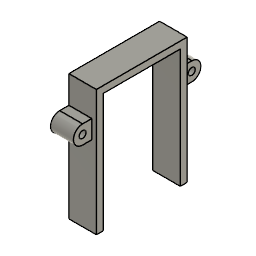
AG05 (Autodesk Fusion 360 design; units mm, degrees)
part number: 2025-10-09-12-51-14-243
Autodesk Fusion 360 part; units mm, degrees
note: some values were not read from the file. Set by a fixed rule: which sketch regions a step uses.
sketch "Boceto1" plane through (0, 0, 0) normal (0, 0, 1) x (1, 0, 0)
  line L0 (-38.0232, 20.8447) -> (47.9768, 20.8447)
  line L1 (47.9768, 20.8447) -> (47.9768, -12.6553)
  line L2 (47.9768, -12.6553) -> (-38.0232, -12.6553)
  line L3 (-38.0232, -12.6553) -> (-38.0232, 20.8447)
  line L4 (-41.0232, 23.8447) -> (50.9768, 23.8447)
  line L5 (50.9768, -15.6553) -> (-41.0232, -15.6553)
  line L6 (-38.0232, 20.8447) -> (-41.0232, 20.8447)
  line L7 (-41.0232, 20.8447) -> (50.9768, 20.8447)
  line L8 (-38.0232, -12.6553) -> (-41.0232, -12.6553)
  line L9 (-41.0232, -15.6553) -> (-41.0232, -12.6553)
  line L10 (-41.0232, 20.8447) -> (-41.0232, 23.8447)
  line L11 (47.9768, -12.6553) -> (50.9768, -12.6553)
  line L12 (50.9768, 23.8447) -> (50.9768, 20.8447)
  line L13 (50.9768, -12.6553) -> (50.9768, -15.6553)
  dimension "d1" = 86
  dimension "d2" = 33.5
  dimension "d3" = 3
  dimension "d4" = 3
  dimension "d5" = 3
  dimension "d6" = 3
  constraint horizontal L0
  constraint vertical L1
  constraint horizontal L2
  constraint vertical L3
  constraint horizontal L4
  constraint vertical L12
  constraint horizontal L5
  constraint vertical L9
  constraint coincident L6.end L9
  constraint perpendicular L6 L9
  constraint perpendicular L7 L12
  constraint perpendicular L8 L9
  constraint collinear L9 L10
  constraint coincident L11.end L12
  constraint perpendicular L11 L12
  constraint collinear L12 L13
  measures "d1" distance of L0.start L0.end
  measures "d2" distance of L0.end L1.end
  measures "d3" distance of L0 L4
  measures "d4" distance of L1 L12
  measures "d5" distance of L2 L5
  measures "d6" distance of L3 L9
extrude "Extruir1" add sketch "Boceto1" along normal blind 51 contours L0 L4 L6 L7 L10 L12 | L2 L5 L8 L9 L11 L13 makes body 1 at (20.3102, 20.8447, 17) makes body 2 at (20.3102, -12.6553, 17)
sketch "Boceto2" plane through (0, 0, 51) normal (0, 0, 1) x (-1, 0, 0)
  line L0 (41.0232, -20.8447) -> (-50.9768, -20.8447)
  line L1 (-50.9768, -20.8447) -> (-50.9768, -23.8447)
  line L2 (-50.9768, -23.8447) -> (41.0232, -23.8447)
  line L3 (41.0232, -23.8447) -> (41.0232, -20.8447)
  line L4 (41.0232, -23.8447) -> (-50.9768, -23.8447)
  line L5 (-50.9768, -23.8447) -> (-50.9768, 15.6553)
  line L6 (-50.9768, 15.6553) -> (41.0232, 15.6553)
  line L7 (41.0232, 15.6553) -> (41.0232, -23.8447)
  dimension "d9" = 39.5
  dimension "d12" = 92
  constraint horizontal L4
  constraint vertical L5
  constraint horizontal L6
  constraint vertical L7
  constraint coincident L2.end L3.start
  measures "d9" distance of L1.end L5.end
  measures "d12" distance of L5 L7
extrude "Extruir2" add sketch "Boceto2" along normal blind 3 bodies 1 2
sketch "Boceto3" plane through (0, 0, 51) normal (0, 0, -1) x (1, 0, 0)
  line L0 (-41.0232, -20.8447) -> (50.9768, -20.8447)
  line L1 (50.9768, -20.8447) -> (50.9768, 12.6553)
  line L2 (50.9768, 12.6553) -> (-41.0232, 12.6553)
  line L3 (-41.0232, 12.6553) -> (-41.0232, -20.8447)
  line L4 (50.9768, 12.6553) -> (47.9768, 12.6553)
  line L5 (47.9768, 12.6553) -> (47.9768, 5.6553)
  line L6 (47.9768, 5.6553) -> (50.9768, 5.6553)
  line L7 (50.9768, 5.6553) -> (50.9768, 12.6553)
  line L8 (50.9768, -20.8447) -> (47.9768, -20.8447)
  line L9 (47.9768, -20.8447) -> (47.9768, -13.8447)
  line L10 (47.9768, -13.8447) -> (50.9768, -13.8447)
  line L11 (50.9768, -13.8447) -> (50.9768, -20.8447)
  dimension "d13" = 3
  dimension "d14" = 3
  dimension "d16" = 7
  dimension "d17" = 7
  constraint horizontal L4
  constraint vertical L5
  constraint horizontal L6
  constraint vertical L7
  constraint coincident L1.end L2.start
  constraint horizontal L8
  constraint vertical L9
  constraint horizontal L10
  constraint vertical L11
  constraint coincident L0.end L1.start
  measures "d13" distance of L5 L7
  measures "d14" distance of L9 L11
  measures "d16" distance of L4.end L5.end
  measures "d17" distance of L0.end L10.end
extrude "Extruir3" add sketch "Boceto3" along normal blind 51 contours L0 L1 L8 L9 L10 L11 | L1 L2 L4 L5 L6 L7 bodies 1
extrude "Extruir4" cut 1 faces at (50.9768, -12.322, 35) along direction (-1, 0, 0) blind 80 on bodies 1 bodies 1
extrude "Extruir5" add 2 faces at (-37.0232, -14.6553, 0) (-37.0232, 22.8447, 0) along direction (0, 0, -1) blind 0.75 on bodies 1 bodies 1
sketch "Boceto4" plane through (0, 0, -0.75) normal (0, 0, -1) x (1, 0, 0)
  line L0 (-29.0232, -23.8447) -> (-29.0232, -20.8447)
  line L1 (-29.0232, -20.8447) -> (-41.0232, -20.8447)
  line L2 (-41.0232, -20.8447) -> (-41.0232, -23.8447)
  line L3 (-41.0232, -23.8447) -> (-29.0232, -23.8447)
  line L4 (-35.0232, -23.8447) -> (-35.0232, -27.8447) construction
  dimension "d24" = 4
  constraint midpoint L3 L4.start
  constraint perpendicular L3 L4
  measures "d24" distance of L4.start L4.end
sketch "Boceto5" plane through (-41.0232, 0, 0) normal (-1, 0, 0) x (0, -1, 0)
  line L0 (-20.8447, -0.75) -> (-20.8447, 51)
  line L1 (-20.8447, 51) -> (12.6553, 51)
  line L2 (12.6553, 51) -> (12.6553, -0.75)
  line L3 (12.6553, -0.75) -> (15.6553, -0.75)
  line L4 (15.6553, -0.75) -> (15.6553, 54)
  line L5 (15.6553, 54) -> (-23.8447, 54)
  line L6 (-23.8447, 54) -> (-23.8447, -0.75)
  line L7 (-23.8447, -0.75) -> (-20.8447, -0.75)
  line L8 (15.6553, -0.75) -> (15.6553, 51) construction
  line L9 (12.6553, -0.75) -> (-20.8447, -0.75) construction
  line L10 (-4.0947, -0.75) -> (-4.0947, 51) construction
  line L11 (-4.0947, 25.125) -> (-4.0947, 51) construction
  line L12 (-4.0947, 38.0625) -> (-23.8447, 38.0625) construction
  line L13 (-4.0947, 38.0625) -> (12.6553, 38.0625) construction
  line L14 (12.6553, 38.0625) -> (19.6553, 38.0625) construction
  line L15 (-23.8447, 38.0625) -> (-27.8447, 38.0625) construction
  circle A0 centre (-27.8447, 38.0625) radius 4
  line L16 (-27.8447, 42.0625) -> (-23.8447, 42.0625)
  line L17 (-27.8447, 34.0625) -> (-23.8447, 34.0625)
  circle A1 centre (-27.8447, 38.0625) radius 1.5
  line L18 (19.6553, 42.0625) -> (15.6553, 42.0625)
  circle A2 centre (19.6553, 38.0625) radius 4
  circle A3 centre (19.6553, 38.0625) radius 1.5
  line L19 (19.6553, 34.0625) -> (15.6553, 34.0625)
  dimension "d25" = 7
  dimension "d26" = 4
  dimension "d27" = 3
  constraint coincident L3.end L4.start
  constraint coincident L4 L8.end
  constraint coincident L2.end L3.start
  constraint coincident L0.start L7.end
  constraint midpoint L9 L10.start
  constraint midpoint L1 L10.end
  constraint midpoint L10 L11.start
  constraint midpoint L11 L12.start
  constraint coincident L6 L12.end
  constraint perpendicular L6 L12
  constraint coincident L2 L13.end
  constraint perpendicular L2 L13
  constraint perpendicular L8 L14
  constraint perpendicular L6 L15
  constraint coincident L15.end A0.centre
  constraint coincident L12.end A0
  constraint coincident A0 L16.start
  constraint coincident L6 L16.end
  constraint tangent A0 L16
  constraint perpendicular L6 L16
  constraint coincident A0 L17.start
  constraint coincident L6 L17.end
  constraint tangent A0 L17
  constraint perpendicular L6 L17
  constraint symmetric L11 A0 A2
  constraint symmetric L11 L16.start L18.start
  constraint symmetric L11 L16.end L18.end
  constraint symmetric L11 L17.start L19.start
  constraint symmetric L11 L17.end L19.end
  constraint symmetric L11 A1 A3
  measures "d25" distance of L13.end L14.end
  measures "d26" distance of L12.end L15.end
  measures "d27" diameter of A1
extrude "Extruir6" add sketch "Boceto5" against normal blind 10 contours L6 A0 L17 | L6 A0 L16 | A0 | L4 A2 L19 | L4 L18 A2 | A2 bodies 1
equation "d12 = 86 mm + 6 mm"
equation "d25 = 3 mm + 4 mm"
named bodies: "AG06"
